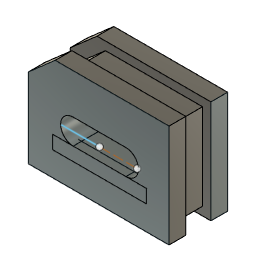
Wii USB C Plug v6 (Autodesk Fusion 360 design; units mm, degrees)
Autodesk Fusion 360 part; units mm, degrees
sketch "Sketch1" plane through (0, 0, 0) normal (0, 1, 0) x (1, 0, 0)
  line L0 (0, 0) -> (0, -7.5)
  line L1 (0, 0) -> (14.8, 0)
  line L2 (14.8, 0) -> (14.8, -10.3)
  line L3 (14.8, -10.3) -> (3.2, -10.3)
  line L4 (0, -7.5) -> (3.2, -10.3)
  dimension "d1" = 14.8
  dimension "d2" = 10.3
  dimension "d3" = 11.6
  constraint coincident L0.start L1.start
  constraint vertical L0
  constraint perpendicular L0 L1
  constraint perpendicular L1 L2
  constraint perpendicular L2 L3
  measures "d1" distance of L0.start L1.end
  measures "d2" distance of L1.end L2.end
  measures "d3" distance of L2.end L3.end
extrude "Extrude1" add sketch "Sketch1" along normal blind 3 makes body 1
sketch "Sketch2" plane through (0, 0, 0) normal (0, -1, 0) x (1, 0, 0)
  line L0 (0, 7.5) -> (0, 0)
  line L1 (0, 0) -> (14.8, 0)
  line L2 (14.8, 0) -> (14.8, 10.3)
  line L3 (14.8, 10.3) -> (3.2, 10.3)
  line L4 (3.2, 10.3) -> (0, 7.5)
  line L5 (-1, -1) -> (15.8, -1)
  line L6 (15.8, -1) -> (15.8, 11.3)
  line L7 (15.8, 11.3) -> (2.2, 11.3)
  line L8 (-1, -1) -> (-1, 8.5)
  line L9 (-1, 8.5) -> (2.2, 11.3)
  dimension "d7" = 16.8
  dimension "d8" = 12.3
  dimension "d9" = 13.6
  dimension "d10" = 9.5
  constraint horizontal L5
  constraint perpendicular L5 L6
  constraint perpendicular L6 L7
  constraint perpendicular L5 L8
  measures "d7" distance of L5.start L5.end
  measures "d8" distance of L5.end L6.end
  measures "d9" distance of L6.end L7.end
  measures "d10" distance of L5.start L8.end
extrude "Extrude2" add sketch "Sketch2" 1 faces at (6, 0, 3.4333) along normal blind 2 contours L0 L1 L2 L3 L4 | L5 L6 L7 L8 L9 on bodies 1 bodies 1
sketch "Sketch3" plane through (0, -2, 0) normal (0, -1, 0) x (1, 0, 0)
  line L0 (-1, -1) -> (15.8, -1)
  line L1 (15.8, -1) -> (15.8, 11.3)
  line L2 (15.8, 11.3) -> (2.2, 11.3)
  line L3 (2.2, 11.3) -> (-1, 8.5)
  line L4 (-1, 8.5) -> (-1, -1)
  line L5 (3, 5) -> (12, 5) construction
  line L6 (3, 5) -> (7.5, 5)
  dimension "d14" = 4.5
  constraint horizontal L5
  constraint parallel L5 L6
  measures "d14" distance of L5.start L6.end
sketch "Sketch4" plane through (0, -2, 0) normal (0, -1, 0) x (1, 0, 0)
sketch "Sketch5" plane through (0, -2, 0) normal (0, -1, 0) x (1, 0, 0)
  line L0 (7.5, 5) -> (12.05, 5)
  line L1 (7.5, 5) -> (2.95, 5)
  line L2 (4.45, 3.5) -> (10.55, 3.5)
  arc A0 (10.55, 3.5) -> (10.55, 6.5) centre (10.55, 5) ccw
  line L3 (10.55, 6.5) -> (4.45, 6.5)
  arc A1 (4.45, 6.5) -> (4.45, 3.5) centre (4.45, 5) ccw
  line L4 (2.95, 5) -> (12.05, 5) construction
  line L5 (7.5, 3.5) -> (13.1, 3.5)
  line L6 (7.5, 3.5) -> (1.9, 3.5)
  line L7 (1.9, 3.5) -> (1.9, 1.9)
  line L8 (1.9, 1.9) -> (13.1, 1.9)
  line L9 (13.1, 1.9) -> (13.1, 3.5)
  dimension "d15" = 4.55
  dimension "d16" = 4.55
  constraint horizontal L0
  constraint parallel L0 L1
  constraint tangent L2 A0
  constraint tangent A0 L3
  constraint parallel L2 L3
  constraint tangent L3 A1
  constraint tangent L2 A1
  constraint midpoint L1.end A1
  constraint midpoint L0.end A0
  constraint midpoint L2 L5.start
  constraint parallel L2 L5
  constraint parallel L2 L6
  constraint perpendicular L6 L7
  constraint perpendicular L7 L8
  constraint perpendicular L5 L9
  measures "d15" distance of L0.start L0.end
  measures "d16" distance of L0.start L1.end
sketch "Sketch6" plane through (0, 3, 0) normal (0, 1, 0) x (-1, 0, 0)
  line L0 (0, 0) -> (0, 7.5)
  line L1 (0, 7.5) -> (-3.2, 10.3)
  line L2 (-3.2, 10.3) -> (-14.8, 10.3)
  line L3 (-14.8, 10.3) -> (-14.8, 0)
  line L4 (-14.8, 0) -> (0, 0)
  line L5 (-15.8, -1) -> (1, -1)
  line L6 (1, -1) -> (1, 8.5)
  line L7 (1, 8.5) -> (-2.2, 11.3)
  line L8 (-2.2, 11.3) -> (-15.8, 11.3)
  line L9 (-15.8, 11.3) -> (-15.8, -1)
  constraint parallel L4 L5
  constraint perpendicular L5 L6
  constraint perpendicular L6 L8
  constraint perpendicular L5 L9
extrude "Extrude3" add sketch "Sketch6" along normal blind 2 contours L0 L1 L2 L3 L4 | L5 L6 L7 L8 L9 bodies 1
sketch "Sketch7" plane through (15.8, 0, 0) normal (1, 0, 0) x (0, 1, 0)
  line L0 (3, 11.3) -> (3, -1)
  line L1 (3, -1) -> (5, -1)
  line L2 (5, -1) -> (5, 11.3)
  line L3 (5, 11.3) -> (3, 11.3)
extrude "Extrude4" add sketch "Sketch5" against normal blind 7 separate body contours L2 L5 L6 L7 L8 L9 makes body 2
extrude "Extrude5" cut 1 faces at (7.5, 5, 2.4333) along direction (0, -1, 0) blind 6 on bodies 2 bodies 1 2
sketch "Sketch8" plane through (0, -2, 0) normal (0, -1, 0) x (1, 0, 0)
  line L0 (7.5, 5) -> (2.95, 5)
  line L1 (7.5, 5) -> (12.05, 5)
  line L2 (4.45, 3.5) -> (10.55, 3.5)
  arc A0 (10.55, 3.5) -> (10.55, 6.5) centre (10.55, 5) ccw
  line L3 (10.55, 6.5) -> (4.45, 6.5)
  arc A1 (4.45, 6.5) -> (4.45, 3.5) centre (4.45, 5) ccw
  line L4 (2.95, 5) -> (12.05, 5) construction
  dimension "d23" = 4.55
  dimension "d24" = 4.55
  constraint horizontal L0
  constraint parallel L0 L1
  constraint tangent L2 A0
  constraint tangent A0 L3
  constraint parallel L2 L3
  constraint tangent L3 A1
  constraint tangent L2 A1
  constraint midpoint L0.end A1
  constraint midpoint L1.end A0
  measures "d23" distance of L0.start L0.end
  measures "d24" distance of L0.start L1.end
extrude "Extrude6" cut sketch "Sketch8" against normal blind 22 bodies 1
sketch "Sketch9" plane through (0, -2, 0) normal (0, -1, 0) x (1, 0, 0)
  line L0 (7.5, 5) -> (12.1, 5)
  line L1 (7.5, 5) -> (2.9, 5)
  line L2 (4.4, 3.5) -> (10.6, 3.5)
  arc A0 (10.6, 3.5) -> (10.6, 6.5) centre (10.6, 5) ccw
  line L3 (10.6, 6.5) -> (4.4, 6.5)
  arc A1 (4.4, 6.5) -> (4.4, 3.5) centre (4.4, 5) ccw
  line L4 (2.9, 5) -> (12.1, 5) construction
  dimension "d27" = 4.6
  dimension "d28" = 4.6
  constraint horizontal L0
  constraint parallel L0 L1
  constraint tangent L2 A0
  constraint tangent A0 L3
  constraint parallel L2 L3
  constraint tangent L3 A1
  constraint tangent L2 A1
  constraint midpoint L1.end A1
  constraint midpoint L0.end A0
  measures "d27" distance of L0.start L0.end
  measures "d28" distance of L0.start L1.end
extrude "Extrude7" cut sketch "Sketch9" against normal blind 17.5 bodies 1
sketch "Sketch10" plane through (0, -2, 0) normal (0, -1, 0) x (1, 0, 0)
  line L0 (7.5, 5) -> (12.15, 5)
  line L1 (7.5, 5) -> (2.85, 5)
  line L2 (4.35, 3.5) -> (10.65, 3.5)
  arc A0 (10.65, 3.5) -> (10.65, 6.5) centre (10.65, 5) ccw
  line L3 (10.65, 6.5) -> (4.35, 6.5)
  arc A1 (4.35, 6.5) -> (4.35, 3.5) centre (4.35, 5) ccw
  line L4 (2.85, 5) -> (12.15, 5) construction
  dimension "d31" = 4.65
  dimension "d32" = 4.65
  constraint horizontal L0
  constraint parallel L0 L1
  constraint tangent L2 A0
  constraint tangent A0 L3
  constraint parallel L2 L3
  constraint tangent L3 A1
  constraint tangent L2 A1
  constraint midpoint L1.end A1
  constraint midpoint L0.end A0
  measures "d31" distance of L0.start L0.end
  measures "d32" distance of L0.start L1.end
extrude "Extrude8" cut sketch "Sketch10" against normal blind 13.6 bodies 1
